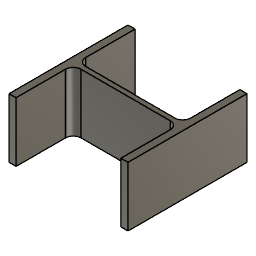
H-200×200×8×12 (Autodesk Fusion 360 design; units mm, degrees)
Autodesk Fusion 360 part; units mm, degrees
sketch "スケッチ1" plane through (0, 0, 0) normal (0, 0, 1) x (1, 0, 0)
  line L0 (0, 100) -> (0, -100)
  line L1 (200, -100) -> (200, 100)
  line L2 (188, -17) -> (188, -100)
  line L3 (12, -100) -> (12, -17)
  line L4 (0, -100) -> (12, -100)
  line L5 (188, -100) -> (200, -100)
  line L6 (12, 17) -> (12, 100)
  line L7 (188, 100) -> (188, 17)
  line L8 (175, 4) -> (25, 4)
  line L9 (25, -4) -> (175, -4)
  arc A0 (25, -4) -> (12, -17) centre (25, -17) ccw
  arc A1 (12, 17) -> (25, 4) centre (25, 17) ccw
  arc A2 (188, -17) -> (175, -4) centre (175, -17) ccw
  arc A3 (175, 4) -> (188, 17) centre (175, 17) ccw
  line L10 (12, 100) -> (0, 100)
  line L11 (200, 100) -> (188, 100)
extrude "押し出し1" add sketch "スケッチ1" along normal blind 100
